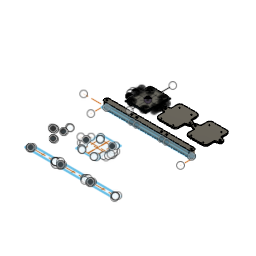
Multi FS40 Bracket v35 (Autodesk Fusion 360 design; units mm, degrees)
Autodesk Fusion 360 part; units mm, degrees
note: some values were not read from the file. Chosen so that the rebuilt part matches the saved one: which face or edge a step refers to. Set by a fixed rule: which sketch regions a step uses.
sketch "Schizzo1" plane through (0, 0, 0) normal (0, 0, 1) x (1, 0, 0)
  line L0 (32, -39) -> (-32, -39)
  line L1 (-32, -39) -> (-32, 39)
  line L2 (-32, 39) -> (32, 39)
  line L3 (32, 39) -> (32, -39)
  line L4 (32, -39) -> (-32, 39) construction
  line L5 (-32, -39) -> (32, 39) construction
  line L6 (-19.25, 24.7) -> (19.25, 24.7) construction
  line L7 (19.25, 24.7) -> (19.25, -33.8) construction
  line L8 (19.25, -33.8) -> (-19.25, -33.8) construction
  line L9 (-19.25, -33.8) -> (-19.25, 24.7) construction
  circle A0 centre (-19.25, 24.7) radius 1.7
  line L10 (0, 0) -> (0, 80) construction
  line L11 (0, 0) -> (0, -60) construction
  line L12 (-32, 0) -> (32, 0) construction
  circle A1 centre (-19.25, -33.8) radius 1.7
  circle A2 centre (19.25, -33.8) radius 1.7
  circle A3 centre (19.25, 24.7) radius 1.7
  line L13 (-32, 0) -> (-48, 0) construction
  line L14 (-40, 20.7498) -> (-40, -19.8726) construction
  circle A4 centre (-40, 0) radius 8
  line L15 (-40, -8) -> (-46, -8) construction
  line L16 (-46, -11.1) -> (-32, -11.1) construction
  arc A5 (-32, -11.1) -> (-40, -8) centre (-40, -19.8726) ccw
  arc A6 (-40, 8) -> (-32, 11.1) centre (-40, 19.8726) ccw
  circle A7 centre (40, 0) radius 8
  arc A8 (32, 11.1) -> (40, 8) centre (40, 19.8726) ccw
  arc A9 (40, -8) -> (32, -11.1) centre (40, -19.8726) ccw
  line L17 (-53.5, -78.6928) -> (226.9, -78.6928)
  line L18 (226.9, -78.6928) -> (226.9, -94.6928)
  line L19 (226.9, -94.6928) -> (-53.5, -94.6928)
  line L20 (-53.5, -94.6928) -> (-53.5, -78.6928)
  circle A10 centre (-45.5, -86.6928) radius 8
  line L21 (-45.5, -78.6928) -> (-45.5, -94.6928) construction
  circle A11 centre (-45.5, -86.6928) radius 2.9
  line L22 (34.5, -78.6928) -> (34.5, -94.6928) construction
  line L23 (226.9, -86.6928) -> (-120, -86.6928) construction
  circle A12 centre (34.5, -86.6928) radius 2.9
  line L24 (50.7, -78.6928) -> (50.7, -94.6928) construction
  circle A13 centre (50.7, -86.6928) radius 2.9
  line L25 (130.7, -78.6928) -> (130.7, -94.6928) construction
  circle A14 centre (130.7, -86.6928) radius 2.9
  line L26 (146.9, -78.6928) -> (146.9, -94.6928) construction
  line L27 (226.9, -78.6928) -> (226.9, -94.6928) construction
  circle A15 centre (146.9, -86.6928) radius 2.9
  circle A16 centre (226.9, -86.6928) radius 2.9
  circle A17 centre (226.9, -86.6928) radius 8
  line L28 (-53.5, -86.6928) -> (234.9, -86.6928)
  line L29 (234.9, -86.6928) -> (-53.5, -86.6928)
  line L30 (-53.5, -86.6928) -> (-53.5, -130) construction
  line L31 (234.9, -86.6928) -> (234.9, -130) construction
  circle A18 centre (-40, 0) radius 3.1
  circle A19 centre (40, 0) radius 3.1
  circle A20 centre (-22, -29) radius 10
  circle A21 centre (22, -29) radius 10
  circle A22 centre (-22, 29) radius 10
  circle A23 centre (22, 29) radius 10
  line L32 (-50, -200) -> (-47, -200)
  line L33 (-47, -200) -> (-47, -206)
  line L34 (-47, -206) -> (-50, -206)
  line L35 (-50, -206) -> (-50, -200)
  circle A24 centre (-50, -203) radius 3
  circle A25 centre (-47, -203) radius 3
  line L36 (20, -171.9) -> (84, -171.9)
  line L37 (84, -171.9) -> (84, -249.9)
  line L38 (84, -249.9) -> (20, -249.9)
  line L39 (20, -249.9) -> (20, -171.9)
  line L40 (20, -210.9) -> (84, -210.9) construction
  circle A26 centre (12, -210.9) radius 3.2
  line L41 (12, -210.9) -> (12, -202.9) construction
  circle A27 centre (12, -207.7) radius 3.2
  line L42 (8.8, -207.7) -> (8.8, -210.9)
  line L43 (15.2, -210.9) -> (15.2, -207.7)
  line L44 (15.2, -210.9) -> (8.8, -210.9) construction
  circle A28 centre (12, -210.9) radius 8
  line L45 (12, -202.9) -> (20, -202.9) construction
  line L46 (20, -202.9) -> (20, -194.9)
  line L47 (20, -194.9) -> (12, -194.9) construction
  line L48 (12, -194.9) -> (12, -202.9) construction
  arc A29 (12, -202.9) -> (20, -194.9) centre (12, -194.9) ccw
  arc A30 (20, -226.9) -> (12, -218.9) centre (12, -226.9) ccw
  line L49 (52, -171.9) -> (52, -249.9) construction
  circle A31 centre (92, -210.9) radius 8
  circle A32 centre (92, -210.9) radius 3.2
  circle A33 centre (92, -207.7) radius 3.2
  line L50 (95.2, -207.7) -> (95.2, -210.9)
  line L51 (88.8, -210.9) -> (88.8, -207.7)
  arc A34 (92, -218.9) -> (84, -226.9) centre (92, -226.9) ccw
  arc A35 (84, -194.9) -> (92, -202.9) centre (92, -194.9) ccw
  circle A36 centre (28, -241.9) radius 8
  circle A37 centre (76, -241.9) radius 8
  circle A38 centre (76, -179.9) radius 8
  circle A39 centre (28, -179.9) radius 8
  line L52 (71.25, -186.2) -> (32.75, -186.2) construction
  line L53 (32.75, -186.2) -> (32.75, -244.7) construction
  line L54 (32.75, -244.7) -> (71.25, -244.7) construction
  line L55 (71.25, -244.7) -> (71.25, -186.2) construction
  line L56 (52, -186.2) -> (52, -244.7) construction
  line L57 (71.25, -215.45) -> (32.75, -215.45) construction
  circle A40 centre (71.25, -186.2) radius 1.7
  circle A41 centre (32.75, -186.2) radius 1.7
  circle A42 centre (71.25, -244.7) radius 1.7
  circle A43 centre (32.75, -244.7) radius 1.7
  circle A44 centre (39.4992, -320.5305) radius 3.1
  line L58 (42.5992, -317.4305) -> (39.4992, -317.4305)
  line L59 (39.4992, -320.5305) -> (39.4992, -317.4305) construction
  line L60 (39.4992, -320.5305) -> (36.3992, -320.5305) construction
  line L61 (42.5992, -323.6305) -> (39.4992, -323.6305)
  line L62 (39.4992, -317.4305) -> (43.2, -317.4305) construction
  line L63 (43.2, -323.6305) -> (39.4992, -323.6305) construction
  line L64 (39.4992, -323.6305) -> (39.4992, -317.4305) construction
  circle A45 centre (42.5992, -320.5305) radius 3.1
  line L65 (127.4992, -312.5305) -> (31.4992, -312.5305)
  line L66 (31.4992, -312.5305) -> (31.4992, -328.5305)
  line L67 (31.4992, -328.5305) -> (127.4992, -328.5305)
  line L68 (127.4992, -328.5305) -> (127.4992, -312.5305)
  line L69 (127.4992, -320.5305) -> (31.4992, -320.5305) construction
  circle A46 centre (119.4992, -320.5305) radius 8
  circle A47 centre (39.4992, -320.5305) radius 8
  line L70 (43.7053, -313.7254) -> (43.7053, -327.3356) construction
  line L71 (12, -207.7) -> (8.8, -207.7) construction
  line L72 (12, -207.7) -> (15.2, -207.7) construction
  line L73 (20, -210.9) -> (-5, -210.9) construction
  circle A48 centre (39.4992, -320.5305) radius 6.2
  circle A49 centre (39.4992, -320.5305) radius 4.1
  circle A50 centre (-47, -203) radius 4
  circle A51 centre (12, -210.9) radius 4.1
  circle A52 centre (92, -210.9) radius 4.1
  line L74 (36.4992, -312.5305) -> (36.4992, -328.5305) construction
  line L75 (36.4992, -315.1046) -> (36.4992, -325.9564)
  line L76 (79.4992, -312.5305) -> (79.4992, -328.5305) construction
  circle A53 centre (119.4992, -320.5305) radius 6.2
  circle A54 centre (116.3992, -320.5305) radius 3.1
  circle A55 centre (119.4992, -320.5305) radius 4.1
  circle A56 centre (119.4992, -320.5305) radius 3.1
  line L77 (122.4992, -315.1046) -> (122.4992, -325.9564)
  circle A57 centre (-46.0282, -223.7668) radius 6
  line L78 (-42.5282, -224.3668) -> (-49.5282, -224.3668)
  line L79 (-49.5282, -224.3668) -> (-49.5282, -223.1668)
  line L80 (-49.5282, -223.1668) -> (-42.5282, -223.1668)
  line L81 (-42.5282, -223.1668) -> (-42.5282, -224.3668)
  line L82 (-42.5282, -224.3668) -> (-49.5282, -223.1668) construction
  line L83 (-49.5282, -224.3668) -> (-42.5282, -223.1668) construction
  line L84 (-46.0282, -223.7668) -> (-46.0282, -217.7668) construction
  line L85 (-46.0282, -223.7668) -> (-46.0282, -229.7668) construction
  line L86 (-46.0282, -223.7668) -> (-40.0282, -223.7668) construction
  line L87 (-46.0282, -223.7668) -> (-52.0282, -223.7668) construction
  circle A58 centre (-46.0282, -223.7668) radius 3
  circle A59 centre (-49.0282, -223.7668) radius 3
  line L88 (-49.0282, -223.7668) -> (-49.0282, -220.7668) construction
  line L89 (-49.0282, -223.7668) -> (-49.0282, -226.7668) construction
  line L90 (-49.0282, -220.7668) -> (-46.0282, -220.7668)
  line L91 (-46.0282, -220.7668) -> (-46.0282, -226.7668)
  line L92 (-46.0282, -226.7668) -> (-49.0282, -226.7668)
  line L93 (-49.0282, -226.7668) -> (-49.0282, -220.7668)
  circle A60 centre (-46.0282, -223.7668) radius 4
  line L94 (138.7992, -317.4305) -> (135.6992, -317.4305)
  line L95 (175.6992, -312.5305) -> (175.6992, -328.5305) construction
  circle A61 centre (135.6992, -320.5305) radius 4.1
  line L96 (138.7992, -323.6305) -> (135.6992, -323.6305)
  line L97 (223.6992, -320.5305) -> (127.6992, -320.5305) construction
  circle A62 centre (135.6992, -320.5305) radius 8
  circle A63 centre (215.6992, -320.5305) radius 4.1
  line L98 (223.6992, -328.5305) -> (223.6992, -312.5305)
  line L99 (223.6992, -312.5305) -> (127.6992, -312.5305)
  circle A64 centre (212.5992, -320.5305) radius 3.1
  line L100 (135.6992, -323.6305) -> (135.6992, -317.4305) construction
  circle A65 centre (135.6992, -320.5305) radius 3.1
  line L101 (135.6992, -320.5305) -> (135.6992, -317.4305) construction
  line L102 (132.6992, -315.1046) -> (132.6992, -325.9564)
  line L103 (135.6992, -317.4305) -> (139.4, -317.4305) construction
  line L104 (139.9053, -313.7254) -> (139.9053, -327.3356) construction
  line L105 (127.6992, -328.5305) -> (223.6992, -328.5305)
  circle A66 centre (138.7992, -320.5305) radius 3.1
  line L106 (218.6992, -315.1046) -> (218.6992, -325.9564)
  line L107 (132.6992, -312.5305) -> (132.6992, -328.5305) construction
  line L108 (139.4, -323.6305) -> (135.6992, -323.6305) construction
  circle A67 centre (215.6992, -320.5305) radius 8
  circle A68 centre (215.6992, -320.5305) radius 6.2
  line L109 (135.6992, -320.5305) -> (132.5992, -320.5305) construction
  circle A69 centre (135.6992, -320.5305) radius 6.2
  circle A70 centre (215.6992, -320.5305) radius 3.1
  line L110 (127.6992, -312.5305) -> (127.6992, -328.5305)
  line L111 (-52.4947, -313.7254) -> (-52.4947, -327.3356) construction
  circle A71 centre (-56.7008, -320.5305) radius 4.1
  line L112 (-53.6008, -317.4305) -> (-56.7008, -317.4305)
  line L113 (-53.6008, -323.6305) -> (-56.7008, -323.6305)
  line L114 (31.2992, -312.5305) -> (-64.7008, -312.5305)
  circle A72 centre (-53.6008, -320.5305) radius 3.1
  circle A73 centre (23.2992, -320.5305) radius 3.1
  line L115 (-56.7008, -317.4305) -> (-53, -317.4305) construction
  line L116 (-59.7008, -312.5305) -> (-59.7008, -328.5305) construction
  line L117 (-64.7008, -328.5305) -> (31.2992, -328.5305)
  line L118 (-53, -323.6305) -> (-56.7008, -323.6305) construction
  line L119 (26.2992, -315.1046) -> (26.2992, -325.9564)
  line L120 (-56.7008, -320.5305) -> (-59.8008, -320.5305) construction
  line L121 (-64.7008, -312.5305) -> (-64.7008, -328.5305)
  line L122 (31.2992, -320.5305) -> (-64.7008, -320.5305) construction
  line L123 (-56.7008, -320.5305) -> (-56.7008, -317.4305) construction
  circle A74 centre (20.1992, -320.5305) radius 3.1
  circle A75 centre (23.2992, -320.5305) radius 4.1
  line L124 (-16.7008, -312.5305) -> (-16.7008, -328.5305) construction
  circle A76 centre (23.2992, -320.5305) radius 6.2
  line L125 (-59.7008, -315.1046) -> (-59.7008, -325.9564)
  circle A77 centre (23.2992, -320.5305) radius 8
  line L126 (31.2992, -328.5305) -> (31.2992, -312.5305)
  line L127 (-56.7008, -323.6305) -> (-56.7008, -317.4305) construction
  line L128 (31.4992, -312.5305) -> (31.4992, -328.5305)
  circle A78 centre (-56.7008, -320.5305) radius 6.2
  circle A79 centre (-56.7008, -320.5305) radius 3.1
  circle A80 centre (-56.7008, -320.5305) radius 8
  line L129 (-64.7008, -312.5305) -> (223.6992, -312.5305)
  line L130 (223.6992, -312.5305) -> (223.6992, -328.5305)
  line L131 (223.6992, -328.5305) -> (-64.7008, -328.5305)
  line L132 (-64.7008, -328.5305) -> (-64.7008, -312.5305)
  circle A81 centre (71.25, -186.2) radius 3
  circle A82 centre (32.75, -186.2) radius 3
  circle A83 centre (71.25, -244.7) radius 3
  circle A84 centre (32.75, -244.7) radius 3
  line L133 (-41, -260.6) -> (-49, -260.6)
  line L134 (-49, -260.6) -> (-49, -259.4)
  line L135 (-49, -259.4) -> (-41, -259.4)
  line L136 (-49, -260.6) -> (-41, -259.4) construction
  circle A85 centre (-45, -260) radius 4
  line L137 (-41, -260.6) -> (-49, -259.4) construction
  line L138 (-43, -260.6) -> (-43, -261.5)
  line L139 (-40.4019, -260) -> (-43, -261.5)
  line L140 (-43, -259.4) -> (-43, -258.5)
  line L141 (-51, -260) -> (-39, -260) construction
  line L142 (-41, -259.4) -> (-41, -260.6)
  line L143 (-43, -256.5359) -> (-43, -263.4641) construction
  line L144 (-40.4019, -260) -> (-43, -258.5)
  circle A86 centre (-45, -260) radius 6
  point P0 (32.75, -186.2)
  point P1 (-46.0282, -223.7668)
  point P2 (-45, -260)
  dimension "d1" = 64
  dimension "d2" = 78
  dimension "d3" = 33.8
  dimension "d5" = 58.5
  dimension "d6" = 19.25
  dimension "d7" = 38.5
  dimension "d8" = 3.4
  dimension "d9" = 3.4
  dimension "d17" = 8
  dimension "d18" = 16
  dimension "d19" = 3.1
  dimension "d20" = 80
  dimension "d21" = 16
  dimension "d22" = 8
  dimension "d23" = 5.8
  dimension "d24" = 80
  dimension "d25" = 5.8
  dimension "d28" = 96.2
  dimension "d29" = 5.8
  dimension "d30" = 80
  dimension "d32" = 5.8
  dimension "d33" = 96.2
  dimension "d34" = 80
  dimension "d35" = 5.8
  dimension "d36" = 5.8
  dimension "d39" = 6.2
  dimension "d87" = 10
  dimension "d88" = 288.4
  dimension "d89" = 3
  dimension "d90" = 6
  dimension "d106" = 64
  dimension "d107" = 78
  dimension "d108" = 6.4
  dimension "d112" = 16
  dimension "d113" = 8
  dimension "d114" = 8
  dimension "d115" = 8
  dimension "d116" = 38.5
  dimension "d117" = 58.5
  dimension "d118" = 3.4
  dimension "d119" = 33.8
  dimension "d122" = 6.2
  dimension "d124" = 96
  dimension "d125" = 16
  dimension "d134" = 12.4
  dimension "d139" = 8.2
  dimension "d140" = 8
  dimension "d142" = 8.2
  dimension "d143" = 3
  dimension "d144" = 80
  dimension "d149" = 12
  dimension "d150" = 7
  dimension "d151" = 1.2
  dimension "d152" = 6
  dimension "d153" = 6
  dimension "d154" = 8
  dimension "d165" = 6.2
  dimension "d166" = 96
  dimension "d167" = 16
  dimension "d168" = 12.4
  dimension "d169" = 8.2
  dimension "d170" = 3
  dimension "d171" = 80
  dimension "d172" = 6.2
  dimension "d173" = 96
  dimension "d174" = 16
  dimension "d175" = 12.4
  dimension "d176" = 8.2
  dimension "d177" = 3
  dimension "d178" = 80
  dimension "d186" = 6
  dimension "d190" = 12
  dimension "d191" = 8
  dimension "d192" = 8
  dimension "d193" = 1.2
  dimension "d194" = 2
  dimension "d195" = 30
  constraint horizontal L0
  constraint perpendicular L0 L1
  constraint parallel L0 L2
  constraint parallel L1 L3
  constraint coincident L4 L10.start
  constraint coincident L5 L10.start
  constraint coincident L10.start L11.start
  constraint horizontal L6
  constraint vertical L7
  constraint horizontal L8
  constraint vertical L9
  constraint coincident L6.start L9.end
  constraint perpendicular L2 L10
  constraint perpendicular L0 L11
  constraint midpoint L1 L12.start
  constraint midpoint L3 L12.end
  constraint coincident L8.end L9.start
  constraint symmetric A0 L11 A3
  constraint symmetric L11 A1 A2
  constraint perpendicular L1 L13
  constraint vertical L14
  constraint coincident A4 L15.start
  constraint coincident L14 L15.start
  constraint tangent A4 L15
  constraint horizontal L16
  constraint coincident L1 L16.end
  constraint coincident L14 A5.centre
  constraint symmetric L13 L15.start A6.start
  constraint symmetric L13 L16.end A6.end
  constraint symmetric L13 A5 A6
  constraint symmetric L10 A4 A7
  constraint symmetric L10 L15.start A9.start
  constraint symmetric L10 L16.end A9.end
  constraint symmetric L10 A5 A9
  constraint symmetric L10 A6.end A8.start
  constraint symmetric L10 A6.start A8.end
  constraint symmetric L10 A6 A8
  constraint horizontal L17
  constraint vertical L18
  constraint horizontal L19
  constraint vertical L20
  constraint tangent L20 A10
  constraint tangent L19 A10
  constraint perpendicular L17 L21
  constraint coincident A10.centre L21
  constraint concentric A10 A11
  constraint perpendicular L19 L22
  constraint midpoint L18 L23.start
  constraint perpendicular L21 L23
  constraint coincident L22 A12.centre
  constraint coincident L23 A12.centre
  constraint perpendicular L19 L24
  constraint coincident L24 A13.centre
  constraint coincident L23 A13.centre
  constraint perpendicular L19 L25
  constraint coincident L25 A14.centre
  constraint coincident L23 A14.centre
  constraint perpendicular L19 L26
  constraint perpendicular L19 L27
  constraint coincident L26 A15.centre
  constraint coincident L23 A15.centre
  constraint coincident L27 L23.start
  constraint coincident L23 A16.centre
  constraint concentric A16 A17
  constraint tangent L17 A17
  constraint midpoint L20 L28.start
  constraint coincident A17 L28.end
  constraint coincident L23 L28.end
  constraint tangent A10 L30
  constraint perpendicular L28 L30
  constraint tangent A17 L31
  constraint coincident L14.end A5.centre
  constraint coincident L13 A4.centre
  constraint concentric A4 A18
  constraint symmetric L10 A18 A19
  constraint tangent L1 A20
  constraint tangent L0 A20
  constraint symmetric L11 A20 A21
  constraint symmetric L12 A20 A22
  constraint symmetric L12 A21 A23
  constraint horizontal L32
  constraint vertical L33
  constraint horizontal L34
  constraint vertical L35
  constraint coincident L34.end A24
  constraint tangent L34 A24
  constraint coincident L32.start A24
  constraint coincident L33.end A25
  constraint coincident L32.end A25
  constraint horizontal L36
  constraint vertical L37
  constraint horizontal L38
  constraint vertical L39
  constraint midpoint L39 L40.start
  constraint midpoint L37 L40.end
  constraint coincident A26.centre L41.start
  constraint perpendicular L36 L41
  constraint coincident L41 A27.centre
  constraint vertical L42
  constraint vertical L43
  constraint tangent A26 L43
  constraint coincident A26 L43.start
  constraint coincident A26 L42.end
  constraint horizontal L44
  constraint coincident L43.start L44.start
  constraint collinear L40 L44
  constraint coincident L40 A26.centre
  constraint tangent L39 A28
  constraint coincident L41.end A28
  constraint horizontal L45
  constraint vertical L46
  constraint horizontal L47
  constraint vertical L48
  constraint tangent L39 A29
  constraint symmetric L40 L41.end A30.end
  constraint symmetric L40 L46.end A30.start
  constraint symmetric L40 A29 A30
  constraint midpoint L36 L49.start
  constraint midpoint L38 L49.end
  constraint symmetric A26 L49 A32
  constraint symmetric L41.end L49 A35.end
  constraint symmetric A27 L49 A33
  constraint symmetric L43.end L49 L51.end
  constraint symmetric L42.start L49 L50.start
  constraint symmetric L42.end L49 L50.end
  constraint symmetric L43.start L49 L51.start
  constraint symmetric A28 L49 A31
  constraint symmetric L46.end L49 A35.start
  constraint symmetric A29 L49 A35
  constraint symmetric A30.end L49 A34.start
  constraint symmetric A30.start L49 A34.end
  constraint symmetric A30 L49 A34
  constraint tangent L38 A36
  constraint tangent L39 A36
  constraint symmetric L49 A36 A37
  constraint symmetric L40 A36 A39
  constraint symmetric L40 A37 A38
  constraint horizontal L52
  constraint vertical L53
  constraint horizontal L54
  constraint vertical L55
  constraint midpoint L52 L56.start
  constraint midpoint L54 L56.end
  constraint midpoint L55 L57.start
  constraint midpoint L53 L57.end
  constraint coincident L52.start L55.end
  constraint symmetric L52.start L56 P0
  constraint symmetric L56 A40 A41
  constraint symmetric L57 A40 A42
  constraint symmetric L57 A41 A43
  constraint collinear L49 L56
  constraint horizontal L58
  constraint tangent A44 L58
  constraint coincident A44.centre L59.start
  constraint coincident A44 L58.end
  constraint vertical L59
  constraint coincident A44 L60.end
  constraint perpendicular L59 L60
  constraint coincident L58.end L59.end
  constraint symmetric L58.start L60 L61.start
  constraint symmetric L58.end L60 L61.end
  constraint horizontal L62
  constraint horizontal L63
  constraint vertical L64
  constraint coincident L61 L63.start
  constraint tangent L58 A45
  constraint tangent L61 A45
  constraint coincident L58.start A45
  constraint horizontal L65
  constraint vertical L66
  constraint horizontal L67
  constraint vertical L68
  constraint midpoint L68 L69.start
  constraint midpoint L66 L69.end
  constraint collinear L60 L69
  constraint tangent L65 A46
  constraint tangent L68 A46
  constraint tangent L67 A46
  constraint tangent L67 A47
  constraint tangent L66 A47
  constraint tangent L65 A47
  constraint coincident A47 L70.start
  constraint coincident A47 L70.end
  constraint perpendicular L67 L70
  constraint tangent L64 A45
  constraint coincident L42 L44.end
  constraint coincident A26.centre A27
  constraint tangent A27 L42
  constraint coincident A27.centre L71.start
  constraint coincident A27 L42.start
  constraint tangent A26 L71
  constraint perpendicular L41 L71
  constraint coincident A27 L43.end
  constraint tangent A26 L72
  constraint parallel L71 L72
  constraint coincident L42.start L71.end
  constraint coincident L42.end L44.end
  constraint coincident L43.end L72.end
  constraint perpendicular L39 L73
  constraint concentric A44 A49
  constraint concentric A25 A50
  constraint concentric A26 A51
  constraint symmetric L49 A51 A52
  constraint coincident L65 L74.start
  constraint coincident L67 L74.end
  constraint perpendicular L67 L74
  constraint coincident A48 L75.start
  constraint coincident L74 L75.start
  constraint coincident A48 L75.end
  constraint coincident L74 L75.end
  constraint midpoint L65 L76.start
  constraint midpoint L67 L76.end
  constraint symmetric A44 L76 A56
  constraint symmetric A45 L76 A54
  constraint symmetric A48 L76 A53
  constraint symmetric A49 L76 A55
  constraint symmetric L75.start L76 L77.start
  constraint symmetric L75.end L76 L77.end
  constraint horizontal L78
  constraint perpendicular L78 L79
  constraint parallel L78 L80
  constraint parallel L79 L81
  constraint coincident L82 P1
  constraint coincident L83 P1
  constraint coincident P1 A57.centre
  constraint coincident A57 L84.end
  constraint vertical L84
  constraint coincident A57 L85.end
  constraint parallel L84 L85
  constraint coincident A57 L86.end
  constraint perpendicular L85 L86
  constraint coincident A57 L87.end
  constraint parallel L78 L87
  constraint midpoint L87 A59.centre
  constraint coincident A59.centre L88.start
  constraint coincident A59 L88.end
  constraint tangent A58 L88
  constraint vertical L88
  constraint coincident A59 L89.end
  constraint tangent A58 L89
  constraint perpendicular L78 L89
  constraint horizontal L90
  constraint vertical L91
  constraint horizontal L92
  constraint vertical L93
  constraint midpoint L85 L91.end
  constraint concentric A57 A60
  constraint horizontal L94
  constraint tangent L94 A65
  constraint coincident A61.centre A62.centre
  constraint coincident L94.end A65
  constraint vertical L101
  constraint coincident L109.end A65
  constraint perpendicular L101 L109
  constraint coincident L94.end L100.end
  constraint symmetric L96.start L94.start L109
  constraint symmetric L96.end L94.end L109
  constraint horizontal L103
  constraint horizontal L108
  constraint vertical L100
  constraint coincident L108.start L96
  constraint tangent L94 A66
  constraint tangent L96 A66
  constraint coincident L94.start A66
  constraint horizontal L99
  constraint vertical L110
  constraint horizontal L105
  constraint vertical L98
  constraint midpoint L97.start L98
  constraint midpoint L97.end L110
  constraint collinear L97 L109
  constraint tangent L99 A67
  constraint tangent L98 A67
  constraint tangent L105 A67
  constraint tangent A62 L105
  constraint tangent A62 L110
  constraint tangent A62 L99
  constraint coincident L104.start A62
  constraint coincident L104.end A62
  constraint perpendicular L104 L105
  constraint tangent L100 A66
  constraint concentric A61 A65
  constraint coincident L107.start L99
  constraint coincident L107.end L105
  constraint perpendicular L105 L107
  constraint coincident L102.start A69
  constraint coincident L102.start L107
  constraint coincident L102.end A69
  constraint coincident L102.end L107
  constraint midpoint L95.start L99
  constraint midpoint L95.end L105
  constraint symmetric L95 A65 A70
  constraint symmetric L95 A64 A66
  constraint symmetric L95 A68 A69
  constraint symmetric L95 A61 A63
  constraint symmetric L106.start L102.start L95
  constraint symmetric L106.end L102.end L95
  constraint horizontal L112
  constraint tangent L112 A79
  constraint coincident A71.centre L120.start
  constraint coincident L112.end A79
  constraint vertical L123
  constraint coincident L120.end A79
  constraint perpendicular L120 L123
  constraint coincident L112.end L115.start
  constraint symmetric L113.start L112.start L120
  constraint symmetric L113.end L112.end L120
  constraint horizontal L115
  constraint horizontal L118
  constraint vertical L127
  constraint coincident L118.start L113
  constraint tangent L112 A72
  constraint tangent L113 A72
  constraint coincident L112.start A72
  constraint horizontal L114
  constraint vertical L121
  constraint horizontal L117
  constraint vertical L126
  constraint midpoint L122.start L126
  constraint midpoint L122.end L121
  constraint collinear L120 L122
  constraint tangent L114 A77
  constraint tangent A77 L126
  constraint tangent L117 A77
  constraint tangent L117 A80
  constraint tangent L121 A80
  constraint tangent L114 A80
  constraint coincident L111.start A80
  constraint coincident L111.end A80
  constraint perpendicular L111 L117
  constraint tangent A72 L127
  constraint concentric A71 A79
  constraint coincident L116.start L114
  constraint coincident L116.end L117
  constraint perpendicular L116 L117
  constraint coincident L125.start A78
  constraint coincident L125.start L116
  constraint coincident L125.end A78
  constraint coincident L125.end L116
  constraint midpoint L124.start L114
  constraint midpoint L124.end L117
  constraint symmetric A73 L124 A79
  constraint symmetric A72 A74 L124
  constraint symmetric L124 A76 A78
  constraint symmetric A71 A75 L124
  constraint symmetric L119.start L125.start L124
  constraint symmetric L119.end L125.end L124
  constraint vertical L128
  constraint horizontal L129
  constraint vertical L130
  constraint horizontal L131
  constraint vertical L132
  constraint concentric A40 A81
  constraint symmetric L49 A81 A82
  constraint symmetric L57 A81 A83
  constraint symmetric L57 A82 A84
  constraint concentric A85 A86
  constraint horizontal L133
  constraint perpendicular L133 L134
  constraint parallel L133 L135
  constraint parallel L134 L142
  constraint coincident P2 L137
  constraint coincident P2 L136
  constraint coincident P2 A85.centre
  constraint coincident L143.start A85
  constraint coincident L143.end A85
  constraint vertical L143
  constraint coincident L141.start A86
  constraint coincident L141.end A86
  constraint parallel L135 L141
  constraint coincident L139.start L141
  constraint coincident L140.end L143
  constraint coincident L140.start L135
  constraint coincident L140.start L143
  constraint perpendicular L135 L140
  constraint symmetric L139.start L144.start L141
  constraint symmetric L140.end L138.end L141
  constraint symmetric L140.start L138.start L141
  constraint coincident L17 L21.start
  constraint coincident L17 L22.start
  constraint coincident L17 L24.start
  constraint coincident L17 L25.start
  constraint coincident L17 L26.start
  constraint coincident L17.end A17
  constraint coincident L19 L24.end
  constraint coincident L19 L25.end
  constraint coincident L19 L22.end
  constraint coincident L19 L21.end
  constraint coincident L19 L26.end
  measures "d1" distance of L1.end L2.end
  measures "d2" distance of L0.end L1.end
  measures "d3" distance of L10.start L8
  measures "d5" distance of L6 L8
  measures "d6" distance of L10.start L9
  measures "d7" distance of L7 L9
  measures "d8" diameter of A0
  measures "d9" diameter of A1
  measures "d17" distance of L1 L14.start
  measures "d18" diameter of A4
  measures "d19" distance of L15 L16
  measures "d20" distance of L14 A7.centre
  measures "d21" distance of L17.start L19.end
  measures "d22" radius of A10
  measures "d23" diameter of A11
  measures "d24" distance of L21 L22
  measures "d25" diameter of A12
  measures "d28" distance of A10.centre L24
  measures "d29" diameter of A13
  measures "d30" distance of L24 L25
  measures "d32" diameter of A14
  measures "d33" distance of L24 L26.end
  measures "d34" distance of L26 L27
  measures "d35" diameter of A15
  measures "d36" diameter of A16
  measures "d39" diameter of A18
  measures "d87" radius of A20
  measures "d88" distance of L30 L31
  measures "d89" distance of L32.start L32.end
  measures "d90" distance of L32.start L34.end
  measures "d106" distance of L37.end L38.end
  measures "d107" distance of L36 L38
  measures "d108" diameter of A26
  measures "d112" diameter of A28
  measures "d113" distance of L41.end L45.end
  measures "d114" distance of L41.end L47.end
  measures "d115" radius of A36
  measures "d116" distance of L52.start P0
  measures "d117" distance of L52.start L54.end
  measures "d118" diameter of A40
  measures "d119" distance of L40 L54
  measures "d122" diameter of A44
  measures "d124" distance of L65.start L65.end
  measures "d125" distance of L65.start L67.end
  measures "d134" diameter of A48
  measures "d139" diameter of A49
  measures "d140" diameter of A50
  measures "d142" diameter of A51
  measures "d143" distance of L64 L74
  measures "d144" distance of A44.centre A46.centre
  measures "d149" diameter of A57
  measures "d150" distance of L79.end L80.end
  measures "d151" distance of L78.end L79.end
  measures "d152" diameter of A58
  measures "d153" diameter of A59
  measures "d154" diameter of A60
  measures "d165" diameter of A65
  measures "d166" distance of L98.end L99.end
  measures "d167" distance of L98.start L98.end
  measures "d168" diameter of A69
  measures "d169" diameter of A61
  measures "d170" distance of L100 L107
  measures "d171" distance of A63.centre A61.centre
  measures "d172" diameter of A79
  measures "d173" distance of L114.start L114.end
  measures "d174" distance of L117.end L114.start
  measures "d175" diameter of A78
  measures "d176" diameter of A71
  measures "d177" distance of L116 L127
  measures "d178" distance of A73.centre A71.centre
  measures "d186" diameter of A81
  measures "d190" diameter of A86
  measures "d191" diameter of A85
  measures "d192" distance of L134.end L135.end
  measures "d193" distance of L134.end L133.end
  measures "d194" distance of L142 L143
  measures "d195" angle of L141 L144
extrude "Estrusione1" add sketch "Schizzo1" along normal blind 4 contours L0 L1 L2 L3 A20 A21 A22 A23 | A21 | A20 | L3 A7 A9 | L3 A7 A8 | A7 | L1 A4 A5 | L1 A4 A6 | A4 | A23 | A22 makes body 1
pattern_linear "Serie R1" count 1 spacing 0 along (0, 1, 0) count 3 spacing 96.2 along (1, 0, 0) of bodies 1 makes body 2 at (102.3333, 0.3426, 0) makes body 3 at (198.5333, 0.3426, 0)
extrude "Estrusione2" add sketch "Schizzo1" along normal blind 20 separate body contours L17 A10 A12 A13 A14 A15 A17 L28 L29 | A10 A11 L28 L29 | A10 A11 L28 L29 | L18 A16 A17 L28 L29 | L18 A16 A17 L28 L29 | L19 A10 A12 A13 A14 A15 A17 L28 L29 | L18 A16 A17 L28 L29 | L18 A16 A17 L28 L29 makes body 4
extrude "Estrusione16" add sketch "Schizzo1" along normal blind 5 separate body contours L36 L37 L38 L39 L46 A36 A37 A38 A39 A81 A82 A83 A84 | A39 A82 | A38 A81 | L39 A28 L46 A29 | A39 A41 A82 | A39 A41 A82 | A38 A40 A81 | A38 A40 A81 | A28 | L37 A31 A35 | L39 A28 A30 | L37 A31 A34 | A31 | A36 A84 | A37 A83 | A37 A83 | A37 A83 | A36 A84 | A36 A84 makes body 5
extrude "Estrusione26" cut sketch "Schizzo1" along normal blind 3.2 from surface at 1.8 contours A39 A41 A82 | A39 A41 A82 | A38 A40 A81 | A38 A40 A81 | A37 A83 | A37 A83 | A36 A84 | A36 A84 picked at (68.8429, -244.5366) picked at (68.7431, -245.6171) picked at (34.7512, -246.4676) picked at (35.1571, -244.5366) bodies 5
extrude "Estrusione17" add sketch "Schizzo1" along normal blind 20 separate body contours A44 A45 | A44 A45 A49 | A44 A45 L75 | A44 L58 A45 A49 | A44 L61 A45 A49 | A44 L58 A49 L75 | L58 A45 A49 | A45 A49 | A44 L61 A49 L75 | L61 A45 A49 | A44 L75 | A44 A49 L75 | L58 A45 A48 A49 L75 | L61 A45 A48 A49 L75 | A48 A49 L75 | L65 L67 A46 A47 L129 L131 | A46 | A47 | A53 A55 L77 | A53 A54 A55 L77 | A53 A54 A55 L77 | A54 A55 | A54 A55 A56 L77 | A55 A56 L77 | A54 A55 A56 L77 | A54 A55 A56 | A54 A56 L77 | A56 L77 | A54 A56 makes body 6
extrude "Estrusione18" cut sketch "Schizzo1" along normal blind 20 contours A44 A45 | A44 A45 A49 | A44 A45 L75 | A44 L58 A45 A49 | A44 L61 A45 A49 | A44 L58 A49 L75 | L58 A45 A49 | A45 A49 | A44 L61 A49 L75 | L61 A45 A49 | A44 L75 | A44 A49 L75 | A54 A55 | A54 A55 A56 L77 | A55 A56 L77 | A54 A55 A56 L77 | A54 A55 A56 | A54 A56 L77 | A56 L77 | A54 A56 bodies 6
extrude "Estrusione19" cut sketch "Schizzo1" along normal blind 4 from surface at 16 contours A44 A45 A49 | A44 L58 A45 A49 | A44 L61 A45 A49 | A44 L58 A49 L75 | L58 A45 A49 | A45 A49 | A44 L61 A49 L75 | L61 A45 A49 | A44 A49 L75 | L58 A45 A48 A49 L75 | L61 A45 A48 A49 L75 | A53 A54 A55 L77 | A53 A54 A55 L77 | A55 A56 L77 bodies 6
pattern_linear "Serie R3" count 3 spacing 96.2 along (1, 0, 0) both ways of "Estrusione17", "Estrusione18", "Estrusione19" makes body 7 at (-3.3675, -312.5305, 6.6667) makes body 8 at (189.0325, -312.5305, 6.6667)
extrude "Estrusione25" add sketch "Schizzo1" along normal blind 20 contours L65 L68 A46 L129 | L68 L110 L129 L131 | L67 L68 A46 L131 | A62 L99 L110 L129 | L65 L66 A47 L128 L129 | A62 L105 L110 L131 | L66 L126 L128 L129 L131 | L66 L67 A47 L128 L131 | L114 A77 L126 L129 | L117 A77 L126 L131 bodies 6 7 8
extrude "Estrusione27" add sketch "Schizzo1" along normal blind 7 separate body contours L133 A85 L139 L142 | L133 A85 L138 L139 | L133 A85 L139 | L139 L142 L144 | A85 L139 L142 | L133 L138 L139 | L133 L135 A85 L139 L144 | L133 L134 A85 | A85 L142 L144 | L134 L135 A85 | L135 A85 L142 L144 | L135 A85 L144 | L135 A85 L140 L144 | L135 L140 L144 | A86 makes body 9
extrude "Estrusione28" cut sketch "Schizzo1" along normal blind 2 contours L139 L142 L144 | L133 L138 L139 | L133 L135 A85 L139 L144 | L135 L140 L144 bodies 9
extrude "Estrusione29" add sketch "Schizzo1" along normal blind 21 from surface at 7 contours L133 A85 L138 L139 | L133 A85 L139 | L133 L138 L139 | L133 L135 A85 L139 L144 | L135 A85 L144 | L135 A85 L140 L144 | L135 L140 L144 bodies 9
sketch "Schizzo10" plane through (0, 0, 28) normal (0, 0, 1) x (-1, 0, 0)
  circle A0 centre (45, 260) radius 4
  line L0 (45, 257) -> (45, 263) construction
  line L1 (39, 263) -> (48, 263) construction
  line L2 (42, 257) -> (42, 263) construction
  line L3 (45, 263) -> (42, 263)
  line L4 (45, 257) -> (42, 257) construction
  line L5 (39, 257) -> (39, 263) construction
  arc A1 (42, 263) -> (42, 257) centre (42, 260) ccw
  line L6 (48, 257) -> (39, 257) construction
  line L7 (45, 257) -> (42, 257)
  line L8 (48, 257) -> (45, 257) construction
  arc A2 (45, 257) -> (45, 263) centre (45, 260) ccw
  line L9 (48, 263) -> (48, 257) construction
  line L10 (42, 257) -> (39, 257) construction
  circle A3 centre (45, 260) radius 4
  line L11 (48, 260) -> (39, 260) construction
  line L12 (41, 260.6) -> (49, 260.6) construction
  line L13 (49, 260.6) -> (49, 259.4) construction
  line L14 (49, 259.4) -> (41, 259.4) construction
  line L15 (41, 259.4) -> (41, 260.6) construction
  line L16 (41, 260.6) -> (49, 259.4) construction
  line L17 (49, 260.6) -> (41, 259.4) construction
  line L18 (43, 256.5359) -> (43, 263.4641) construction
  line L19 (43, 258.55) -> (40.4885, 260)
  line L20 (43, 258.55) -> (40.1, 258.55) construction
  line L21 (48, 260) -> (48, 259.4)
  line L22 (48, 259.4) -> (43, 259.4)
  line L23 (43, 259.4) -> (43, 258.55)
  line L24 (48, 260) -> (48, 260.6)
  line L25 (43, 260.6) -> (43, 261.45)
  line L26 (43, 261.45) -> (40.4885, 260)
  line L27 (48, 260.6) -> (43, 260.6)
  point P0 (45, 260)
  point P1 (45, 260)
  point P2 (45, 260)
  dimension "d209" = 9
  dimension "d210" = 6
  dimension "d211" = 8
  dimension "d212" = 1.2
  dimension "d214" = 2
  dimension "d215" = 30
  constraint horizontal L6
  constraint vertical L5
  constraint horizontal L1
  constraint vertical L9
  constraint midpoint L11.start L9
  constraint midpoint L11.end L5
  constraint coincident L0.start L6
  constraint coincident L0.end L1
  constraint perpendicular L0 L1
  constraint coincident L2.start L6
  constraint coincident L2.end L1
  constraint perpendicular L1 L2
  constraint equal L8 L10
  constraint equal L4 L8
  constraint midpoint P2 L0
  constraint midpoint A1.centre L2
  constraint coincident P2 P1
  constraint horizontal L12
  constraint perpendicular L12 L13
  constraint parallel L12 L14
  constraint parallel L13 L15
  constraint coincident L16 P2
  constraint coincident L17 P2
  constraint coincident A3 L18.start
  constraint coincident A3 L18.end
  constraint perpendicular L1 L18
  constraint horizontal L20
  constraint coincident L18 L19.start
  constraint coincident L11 L19.end
  constraint coincident L9 L21.end
  constraint coincident L14 L21.end
  constraint coincident L18 L22.end
  constraint coincident L14 L22.end
  constraint symmetric L21.start L11 L24.start
  constraint symmetric L11 L19.start L25.end
  constraint symmetric L11 L19.end L26.end
  constraint symmetric L11 L21.end L24.end
  constraint symmetric L11 L22.end L25.start
  measures "d209" distance of L6.start L5.start
  measures "d210" distance of L6.start L1.end
  measures "d211" distance of L13.end L14.end
  measures "d212" distance of L12.end L13.end
  measures "d214" distance of L15 L18
  measures "d215" angle of L19 L20
extrude "Estrusione30" add sketch "Schizzo10" along normal blind 4 bodies 9
extrude "Estrusione31" cut sketch "Schizzo10" along normal blind 2 from surface at 2 contours A0 A2 A3 L19 L22 L23 L25 L26 L27 | A0 A3 L19 L26 bodies 9
hidden bodies 5 6 9
equation "d6 = 38.50 mm / 2"
named bodies: "Basetta 1", "Basetta 2", "Basetta 3", "Trave", "BasettaQDS-1", "TraveQDS", "TraveQDS (1)", "TraveQDS (2)", "Mounting Screw V3"
